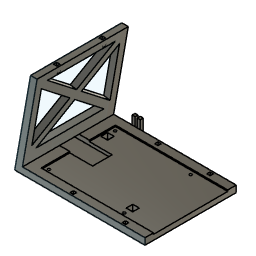
WRO raspberry PI (1) (Autodesk Fusion 360 design; units mm, degrees)
Autodesk Fusion 360 part; units mm, degrees
note: some values were not read from the file. Set by a fixed rule: which sketch regions a step uses.
sketch "Sketch1" plane through (0, 0, 0) normal (0, 1, 0) x (1, 0, 0)
  line L0 (0, 0) -> (12.1554, -68.9365)
  line L1 (0, 0) -> (70, 0) construction
  line L2 (0, 0) -> (100, 0)
  line L3 (100, 0) -> (100, -5)
  line L4 (100, -5) -> (0.8816, -5)
  line L5 (6.0777, -34.4683) -> (10.7761, -32.7582)
  line L6 (6.0777, -34.4683) -> (11.0777, -34.4683) construction
  line L7 (4.1331, -23.4398) -> (8.8315, -21.7297)
  line L8 (4.1331, -23.4398) -> (9.1331, -23.4398) construction
  line L9 (8.8315, -21.7297) -> (10.7761, -32.7582)
  line L10 (10.7761, -32.7582) -> (5, 0)
  line L11 (5, 0) -> (16.8803, -67.3767)
  line L12 (12.1554, -68.9365) -> (20.8902, -68.9365)
  line L13 (16.8803, -67.3767) -> (17.1554, -68.9365)
  dimension "d1" = 70
  dimension "d2" = 80
  dimension "d3" = 100
  dimension "d4" = 5
  dimension "d5" = 5
  dimension "d6" = 20
  dimension "d7" = 20
  dimension "d8" = 5
  constraint horizontal L1
  constraint coincident L0.start L1.start
  constraint parallel L1 L2
  constraint perpendicular L2 L3
  constraint coincident L0 L4.end
  constraint perpendicular L3 L4
  constraint horizontal L6
  constraint midpoint L0 L5.start
  constraint horizontal L8
  constraint coincident L0 L7.start
  constraint coincident L2 L10.end
  constraint parallel L10 L11
  constraint horizontal L12
  constraint coincident L12 L13.end
  constraint parallel L11 L13
  measures "d1" distance of L0.start L0.end
  measures "d2" angle of L0 L1
  measures "d3" distance of L0.start L2.end
  measures "d4" distance of L2.end L3.end
  measures "d5" distance of L5.start L5.end
  measures "d6" angle of L5 L6
  measures "d7" angle of L7 L8
  measures "d8" distance of L7.start L7.end
extrude "Extrude1" add sketch "Sketch1" along normal blind 70 makes body 1
sketch "Sketch2" plane through (0, 0, 0) normal (0, 0, -1) x (1, 0, 0)
  line L0 (100, 0) -> (0, 0)
  line L1 (0, 0) -> (0, -70)
  line L2 (0, -70) -> (100, -70)
  line L3 (100, -70) -> (100, 0)
  line L4 (0, 0) -> (1.25, 0)
  line L5 (1.25, 0) -> (1.25, -1.25)
  line L6 (1.25, -1.25) -> (0, -1.25)
  line L7 (0, -1.25) -> (0, 0)
  line L8 (1.25, -1.25) -> (3.55, -1.25)
  line L9 (3.55, -1.25) -> (3.55, -3.55)
  line L10 (3.55, -3.55) -> (1.25, -3.55)
  line L11 (1.25, -3.55) -> (1.25, -1.25)
  line L12 (0, -70) -> (1.25, -70)
  line L13 (1.25, -70) -> (1.25, -68.75)
  line L14 (1.25, -68.75) -> (0, -68.75)
  line L15 (0, -68.75) -> (0, -70)
  line L16 (1.25, -68.75) -> (3.55, -68.75)
  line L17 (3.55, -68.75) -> (3.55, -66.45)
  line L18 (3.55, -66.45) -> (1.25, -66.45)
  line L19 (1.25, -66.45) -> (1.25, -68.75)
  dimension "d11" = 1.25
  dimension "d12" = 1.25
  dimension "d13" = 2.3
  dimension "d14" = 2.3
  dimension "d15" = 1.25
  dimension "d16" = 1.25
  dimension "d17" = 2.3
  dimension "d18" = 2.3
  constraint horizontal L4
  constraint vertical L5
  constraint horizontal L6
  constraint vertical L7
  constraint coincident L0.end L1.start
  constraint horizontal L8
  constraint vertical L9
  constraint horizontal L10
  constraint vertical L11
  constraint horizontal L12
  constraint vertical L13
  constraint horizontal L14
  constraint vertical L15
  constraint coincident L1.end L2.start
  constraint horizontal L16
  constraint vertical L17
  constraint horizontal L18
  constraint vertical L19
  measures "d11" distance of L0.end L4.end
  measures "d12" distance of L0.end L6.end
  measures "d13" distance of L5.end L8.end
  measures "d14" distance of L5.end L10.end
  measures "d15" distance of L1.end L12.end
  measures "d16" distance of L1.end L14.end
  measures "d17" distance of L13.end L16.end
  measures "d18" distance of L13.end L18.end
extrude "Extrude2" add sketch "Sketch2" along normal blind 5 contours L8 L9 L10 L11 | L16 L17 L18 L19 bodies 1
sketch "Sketch3" plane through (0, 0, 5) normal (0, 0, 1) x (-1, 0, 0)
  line L0 (-5.8816, 0) -> (-100, 0)
  line L1 (-100, 0) -> (-100, -70)
  line L2 (-100, -70) -> (-5.8816, -70)
  line L3 (-5.8816, -70) -> (-5.8816, 0)
  line L4 (-100, 0) -> (-100, -35)
  line L5 (-100, -35) -> (-100, -6.5)
  line L6 (-100, -6.5) -> (-13.75, -6.5)
  line L7 (-13.75, -6.5) -> (-13.75, -63.5)
  line L8 (-13.75, -63.5) -> (-100, -63.5)
  line L9 (-100, -63.5) -> (-100, -6.5)
  dimension "d21" = 35
  dimension "d22" = 28.5
  dimension "d23" = 86.25
  dimension "d24" = 57
  constraint coincident L0.end L1.start
  constraint perpendicular L0 L4
  constraint parallel L4 L5
  constraint horizontal L6
  constraint vertical L7
  constraint horizontal L8
  constraint vertical L9
  measures "d21" distance of L0.end L4.end
  measures "d22" distance of L4.end L5.end
  measures "d23" distance of L5.end L6.end
  measures "d24" distance of L5.end L8.end
extrude "Extrude3" cut sketch "Sketch3" against normal blind 1 contours L1 L4 L5 L6 L7 L8 L9 bodies 1
sketch "Sketch4" plane through (0, 0, 4) normal (0, 0, 1) x (-1, 0, 0)
  line L0 (-100, -63.5) -> (-13.75, -63.5)
  line L1 (-13.75, -63.5) -> (-13.75, -6.5)
  line L2 (-13.75, -6.5) -> (-100, -6.5)
  line L3 (-100, -6.5) -> (-100, -63.5)
  line L4 (-13.75, -6.5) -> (-13.75, -28.5)
  line L5 (-13.75, -28.5) -> (-31.25, -28.5)
  line L6 (-31.25, -28.5) -> (-31.25, -43.5)
  line L7 (-31.25, -43.5) -> (-13.75, -43.5)
  line L8 (-13.75, -43.5) -> (-13.75, -28.5)
  dimension "d27" = 22
  dimension "d28" = 17.5
  dimension "d29" = 15
  constraint coincident L1.end L2.start
  constraint perpendicular L2 L4
  constraint horizontal L5
  constraint vertical L6
  constraint horizontal L7
  constraint vertical L8
  measures "d27" distance of L1.end L4.end
  measures "d28" distance of L4.end L5.end
  measures "d29" distance of L4.end L7.end
extrude "Extrude4" cut sketch "Sketch4" against normal blind 2.5 contours L1 L5 L6 L7 L8 bodies 1
sketch "Sketch5" plane through (13.75, 0, 0) normal (1, 0, 0) x (0, 1, 0)
  line L0 (63.5, 5) -> (6.5, 5)
  line L1 (6.5, 5) -> (6.5, 4)
  line L2 (6.5, 4) -> (28.5, 4)
  line L3 (28.5, 4) -> (28.5, 1.5)
  line L4 (28.5, 1.5) -> (43.5, 1.5)
  line L5 (43.5, 1.5) -> (43.5, 4)
  line L6 (43.5, 4) -> (63.5, 4)
  line L7 (63.5, 4) -> (63.5, 5)
  line L8 (28.5, 1.5) -> (43.5, 1.5)
  line L9 (43.5, 1.5) -> (43.5, 5)
  line L10 (43.5, 5) -> (28.5, 5)
  line L11 (28.5, 5) -> (28.5, 1.5)
  dimension "d32" = 3.5
  constraint horizontal L8
  constraint vertical L9
  constraint horizontal L10
  constraint vertical L11
  constraint coincident L3.end L4.start
  measures "d32" distance of L3.end L10.end
extrude "Extrude5" cut sketch "Sketch5" against normal blind 1000 contours L0 L3 L4 L5 L8 L9 L10 L11 bodies 1
sketch "Sketch6" plane through (0, 0, 4) normal (0, 0, 1) x (-1, 0, 0)
  line L0 (-13.75, -43.5) -> (-31.25, -43.5)
  line L1 (-31.25, -43.5) -> (-31.25, -28.5)
  line L2 (-31.25, -28.5) -> (-13.75, -28.5)
  line L3 (-13.75, -28.5) -> (-13.75, -6.5)
  line L4 (-13.75, -6.5) -> (-100, -6.5)
  line L5 (-100, -6.5) -> (-100, -63.5)
  line L6 (-100, -63.5) -> (-13.75, -63.5)
  line L7 (-13.75, -63.5) -> (-13.75, -43.5)
  line L8 (-13.75, -63.5) -> (-16.55, -63.5)
  line L9 (-16.55, -63.5) -> (-16.55, -60.5)
  circle A0 centre (-16.55, -60.5) radius 1
  dimension "d35" = 2.8
  dimension "d36" = 3
  dimension "d37" = 2
  constraint coincident L6.end L7.start
  constraint perpendicular L7 L8
  constraint perpendicular L6 L9
  constraint coincident L9.end A0.centre
  measures "d35" distance of L6.end L8.end
  measures "d36" distance of L8.end L9.end
  measures "d37" diameter of A0
extrude "Extrude6" cut sketch "Sketch6" against normal blind 67 contours A0 bodies 1
sketch "Sketch7" plane through (0, 0, 4) normal (0, 0, 1) x (-1, 0, 0)
  circle A0 centre (-16.55, -60.5) radius 1
  line L0 (-13.75, -43.5) -> (-31.25, -43.5)
  line L1 (-31.25, -43.5) -> (-31.25, -28.5)
  line L2 (-31.25, -28.5) -> (-13.75, -28.5)
  line L3 (-13.75, -28.5) -> (-13.75, -6.5)
  line L4 (-13.75, -6.5) -> (-100, -6.5)
  line L5 (-100, -6.5) -> (-100, -63.5)
  line L6 (-100, -63.5) -> (-13.75, -63.5)
  line L7 (-13.75, -63.5) -> (-13.75, -43.5)
  line L8 (-16.55, -60.5) -> (-16.55, -59.5)
  line L9 (-16.55, -59.5) -> (-16.55, -56.5)
  line L10 (-16.55, -56.5) -> (-14.75, -56.5)
  line L11 (-14.75, -56.5) -> (-19.75, -56.5)
  line L12 (-19.75, -56.5) -> (-19.75, -51.5)
  line L13 (-19.75, -51.5) -> (-14.75, -51.5)
  line L14 (-14.75, -51.5) -> (-14.75, -56.5)
  dimension "d40" = 3
  dimension "d41" = 1.8
  dimension "d42" = 5
  dimension "d43" = 5
  constraint coincident A0.centre L8.start
  constraint coincident A0 L8.end
  constraint vertical L8
  constraint parallel L8 L9
  constraint perpendicular L7 L10
  constraint horizontal L11
  constraint vertical L12
  constraint horizontal L13
  constraint vertical L14
  measures "d40" distance of L8.end L9.end
  measures "d41" distance of L9.end L10.end
  measures "d42" distance of L10.end L11.end
  measures "d43" distance of L10.end L13.end
extrude "Extrude7" cut sketch "Sketch7" against normal blind 56 contours L10 L11 L12 L13 L14 bodies 1
sketch "Sketch8" plane through (0, 0, 4) normal (0, 0, 1) x (-1, 0, 0)
  line L0 (-19.75, -56.5) -> (-19.75, -51.5)
  line L1 (-19.75, -51.5) -> (-14.75, -51.5)
  line L2 (-14.75, -51.5) -> (-14.75, -56.5)
  line L3 (-14.75, -56.5) -> (-19.75, -56.5)
  circle A0 centre (-16.55, -60.5) radius 1
  line L4 (-13.75, -43.5) -> (-31.25, -43.5)
  line L5 (-31.25, -43.5) -> (-31.25, -28.5)
  line L6 (-31.25, -28.5) -> (-13.75, -28.5)
  line L7 (-13.75, -28.5) -> (-13.75, -6.5)
  line L8 (-13.75, -6.5) -> (-100, -6.5)
  line L9 (-100, -6.5) -> (-100, -63.5)
  line L10 (-100, -63.5) -> (-13.75, -63.5)
  line L11 (-13.75, -63.5) -> (-13.75, -43.5)
  line L12 (-13.75, -6.5) -> (-16.75, -6.5)
  line L13 (-16.75, -6.5) -> (-16.75, -9.5)
  circle A1 centre (-16.75, -9.5) radius 1
  dimension "d46" = 3
  dimension "d47" = 3
  dimension "d48" = 2
  constraint coincident L7.end L8.start
  constraint perpendicular L7 L12
  constraint perpendicular L12 L13
  constraint coincident L13.end A1.centre
  measures "d46" distance of L7.end L12.end
  measures "d47" distance of L12.end L13.end
  measures "d48" diameter of A1
extrude "Extrude8" cut sketch "Sketch8" against normal blind 45 contours A1 bodies 1
sketch "Sketch9" plane through (0, 0, 4) normal (0, 0, 1) x (-1, 0, 0)
  circle A0 centre (-16.75, -9.5) radius 1
  line L0 (-19.75, -56.5) -> (-19.75, -51.5)
  line L1 (-19.75, -51.5) -> (-14.75, -51.5)
  line L2 (-14.75, -51.5) -> (-14.75, -56.5)
  line L3 (-14.75, -56.5) -> (-19.75, -56.5)
  circle A1 centre (-16.55, -60.5) radius 1
  line L4 (-13.75, -43.5) -> (-31.25, -43.5)
  line L5 (-31.25, -43.5) -> (-31.25, -28.5)
  line L6 (-31.25, -28.5) -> (-13.75, -28.5)
  line L7 (-13.75, -28.5) -> (-13.75, -6.5)
  line L8 (-13.75, -6.5) -> (-100, -6.5)
  line L9 (-100, -6.5) -> (-100, -63.5)
  line L10 (-100, -63.5) -> (-13.75, -63.5)
  line L11 (-13.75, -63.5) -> (-13.75, -43.5)
  line L12 (-16.55, -60.5) -> (-74.55, -60.5)
  circle A2 centre (-74.55, -60.5) radius 1
  line L13 (-74.55, -60.5) -> (-74.55, -9.5)
  circle A3 centre (-74.55, -9.5) radius 1
  dimension "d51" = 58
  dimension "d52" = 2
  dimension "d53" = 51
  dimension "d54" = 2
  constraint coincident A1.centre L12.start
  constraint perpendicular L11 L12
  constraint coincident L12.end A2.centre
  constraint vertical L13
  constraint coincident L13.end A3.centre
  measures "d51" distance of A1.centre L12.end
  measures "d52" diameter of A2
  measures "d53" distance of L12.end L13.end
  measures "d54" diameter of A3
extrude "Extrude9" cut sketch "Sketch9" against normal blind 5 contours L12 A2 L13 | L12 A2 L13 | A3 bodies 1
sketch "Sketch10" plane through (0, 0, 4) normal (0, 0, 1) x (-1, 0, 0)
  circle A0 centre (-74.55, -60.5) radius 1
  circle A1 centre (-74.55, -9.5) radius 1
  circle A2 centre (-16.75, -9.5) radius 1
  line L0 (-19.75, -56.5) -> (-19.75, -51.5)
  line L1 (-19.75, -51.5) -> (-14.75, -51.5)
  line L2 (-14.75, -51.5) -> (-14.75, -56.5)
  line L3 (-14.75, -56.5) -> (-19.75, -56.5)
  circle A3 centre (-16.55, -60.5) radius 1
  line L4 (-13.75, -43.5) -> (-31.25, -43.5)
  line L5 (-31.25, -43.5) -> (-31.25, -28.5)
  line L6 (-31.25, -28.5) -> (-13.75, -28.5)
  line L7 (-13.75, -28.5) -> (-13.75, -6.5)
  line L8 (-13.75, -6.5) -> (-100, -6.5)
  line L9 (-100, -6.5) -> (-100, -63.5)
  line L10 (-100, -63.5) -> (-13.75, -63.5)
  line L11 (-13.75, -63.5) -> (-13.75, -43.5)
  line L12 (-74.55, -9.5) -> (-74.55, -13.5)
  line L13 (-74.55, -13.5) -> (-77.05, -13.5)
  line L14 (-77.05, -13.5) -> (-77.05, -18.5)
  line L15 (-77.05, -18.5) -> (-74.55, -18.5)
  line L16 (-74.55, -18.5) -> (-74.55, -13.5)
  line L17 (-77.05, -18.5) -> (-72.05, -18.5)
  line L18 (-72.05, -18.5) -> (-72.05, -13.5)
  line L19 (-72.05, -13.5) -> (-77.05, -13.5)
  line L20 (-77.05, -13.5) -> (-77.05, -18.5)
  dimension "d57" = 4
  dimension "d58" = 2.5
  dimension "d59" = 5
  dimension "d60" = 5
  dimension "d61" = 5
  constraint coincident A1.centre L12.start
  constraint vertical L12
  constraint horizontal L13
  constraint vertical L14
  constraint horizontal L15
  constraint vertical L16
  constraint horizontal L17
  constraint vertical L18
  constraint horizontal L19
  constraint vertical L20
  measures "d57" distance of A1.centre L12.end
  measures "d58" distance of L12.end L13.end
  measures "d59" distance of L12.end L15.end
  measures "d60" distance of L14.end L17.end
  measures "d61" distance of L14.end L13.end
extrude "Extrude10" cut sketch "Sketch10" against normal blind 5 contours L13 L14 L15 L16 L17 L19 L20 | L16 L17 L18 L19 bodies 1
sketch "Sketch11" plane through (0, 0, 0) normal (-0.984808, 0, 0.173648) x (0, -1, 0)
  line L0 (-28.5, 1.5231) -> (-43.5, 1.5231)
  line L1 (-43.5, 1.5231) -> (-43.5, 5.0771)
  line L2 (-43.5, 5.0771) -> (-28.5, 5.0771)
  line L3 (-28.5, 5.0771) -> (-28.5, 1.5231)
  line L4 (0, 0) -> (0, 70)
  line L5 (0, 70) -> (-70, 70)
  line L6 (-70, 70) -> (-70, 0)
  line L7 (-70, 0) -> (0, 0)
sketch "Sketch12" plane through (0, 0, 0) normal (-0.984808, 0, 0.173648) x (0, -1, 0)
  line L0 (-70, 70) -> (0, 70)
  line L1 (0, 70) -> (0, 10)
  line L2 (0, 10) -> (-70, 10)
  line L3 (-70, 10) -> (-70, 70)
  line L4 (-70, 70) -> (-65, 70)
  line L5 (-65, 70) -> (-65, 65)
  line L6 (-65, 65) -> (-5, 65)
  line L7 (-5, 65) -> (-5, 15)
  line L8 (-5, 15) -> (-65, 15)
  line L9 (-65, 15) -> (-65, 65)
  line L10 (-65, 15) -> (-65, 19)
  line L11 (-65, 15) -> (-61, 15)
  line L12 (-5, 65) -> (-9, 65)
  line L13 (-5, 65) -> (-5, 61)
  line L14 (-65, 19) -> (-9, 65)
  line L15 (-5, 61) -> (-61, 15)
  line L16 (-65, 65) -> (-65, 61)
  line L17 (-65, 65) -> (-61, 65)
  line L18 (-5, 15) -> (-5, 19)
  line L19 (-5, 15) -> (-9, 15)
  line L20 (-9, 15) -> (-65, 61)
  line L21 (-5, 19) -> (-61, 65)
  dimension "d64" = 70
  dimension "d65" = 60
  dimension "d66" = 5
  dimension "d67" = 5
  dimension "d68" = 60
  dimension "d69" = 50
  dimension "d70" = 4
  dimension "d71" = 4
  dimension "d72" = 4
  dimension "d73" = 4
  dimension "d74" = 4
  dimension "d75" = 4
  dimension "d76" = 4
  dimension "d77" = 4
  constraint horizontal L0
  constraint vertical L1
  constraint horizontal L2
  constraint vertical L3
  constraint perpendicular L3 L4
  constraint perpendicular L4 L5
  constraint horizontal L6
  constraint vertical L7
  constraint horizontal L8
  constraint vertical L9
  constraint perpendicular L8 L10
  constraint perpendicular L10 L11
  constraint coincident L6 L12.end
  constraint perpendicular L6 L13
  constraint perpendicular L6 L16
  constraint perpendicular L16 L17
  constraint perpendicular L8 L18
  constraint perpendicular L18 L19
  measures "d64" distance of L0.start L0.end
  measures "d65" distance of L0.start L2.end
  measures "d66" distance of L0.start L4.end
  measures "d67" distance of L4.end L5.end
  measures "d68" distance of L5.end L6.end
  measures "d69" distance of L5.end L8.end
  measures "d70" distance of L8.end L10.end
  measures "d71" distance of L8.end L11.end
  measures "d72" distance of L6.end L12.end
  measures "d73" distance of L6.end L13.end
  measures "d74" distance of L5.end L16.end
  measures "d75" distance of L5.end L17.end
  measures "d76" distance of L7.end L18.end
  measures "d77" distance of L7.end L19.end
extrude "Extrude11" cut sketch "Sketch12" against normal blind 5 contours L6 L14 L21 | L9 L14 L20 | L7 L15 L21 | L8 L15 L20 bodies 1
sketch "Sketch13" plane through (0, 0, 68.9365) normal (0, 0, 1) x (-1, 0, 0)
  line L0 (-12.1554, 0) -> (-17.1554, 0)
  line L1 (-17.1554, 0) -> (-17.1554, -70)
  line L2 (-17.1554, -70) -> (-12.1554, -70)
  line L3 (-12.1554, -70) -> (-12.1554, 0)
  line L4 (-12.1554, 0) -> (-12.1554, -35)
  line L5 (-12.1554, -35) -> (-12.1554, -15)
  line L6 (-12.1554, -15) -> (-12.1554, -55)
  line L7 (-12.1554, -55) -> (-17.1554, -55)
  line L8 (-17.1554, -55) -> (-17.1554, -15)
  line L9 (-17.1554, -15) -> (-12.1554, -15)
  line L10 (-12.1554, -15) -> (-12.1554, -55)
  line L11 (-17.1554, -55) -> (-17.1554, -53.65)
  line L12 (-17.1554, -53.65) -> (-15.8054, -53.65)
  line L13 (-15.8054, -53.65) -> (-13.5054, -53.65)
  line L14 (-13.5054, -53.65) -> (-13.5054, -51.35)
  line L15 (-13.5054, -51.35) -> (-15.8054, -51.35)
  line L16 (-15.8054, -51.35) -> (-15.8054, -53.65)
  line L17 (-12.1554, -15) -> (-12.1554, -16.35)
  line L18 (-12.1554, -16.35) -> (-13.5054, -16.35)
  line L19 (-13.5054, -16.35) -> (-15.8054, -16.35)
  line L20 (-15.8054, -16.35) -> (-15.8054, -18.65)
  line L21 (-15.8054, -18.65) -> (-13.5054, -18.65)
  line L22 (-13.5054, -18.65) -> (-13.5054, -16.35)
  dimension "d80" = 35
  dimension "d81" = 20
  dimension "d82" = 40
  dimension "d83" = 5
  dimension "d84" = 40
  dimension "d85" = 1.35
  dimension "d86" = 1.35
  dimension "d87" = 2.3
  dimension "d88" = 2.3
  dimension "d89" = 1.35
  dimension "d90" = 1.35
  dimension "d91" = 2.3
  dimension "d92" = 2.3
  constraint coincident L0.start L3.end
  constraint perpendicular L2 L4
  constraint parallel L4 L5
  constraint parallel L3 L6
  constraint horizontal L7
  constraint vertical L8
  constraint horizontal L9
  constraint vertical L10
  constraint perpendicular L7 L11
  constraint perpendicular L8 L12
  constraint horizontal L13
  constraint vertical L14
  constraint horizontal L15
  constraint vertical L16
  constraint parallel L6 L17
  constraint perpendicular L5 L18
  constraint horizontal L19
  constraint vertical L20
  constraint horizontal L21
  constraint vertical L22
  measures "d80" distance of L0.start L4.end
  measures "d81" distance of L4.end L5.end
  measures "d82" distance of L5.end L6.end
  measures "d83" distance of L6.end L7.end
  measures "d84" distance of L6.end L5.end
  measures "d85" distance of L7.end L11.end
  measures "d86" distance of L11.end L12.end
  measures "d87" distance of L12.end L13.end
  measures "d88" distance of L12.end L15.end
  measures "d89" distance of L5.end L17.end
  measures "d90" distance of L17.end L18.end
  measures "d91" distance of L18.end L19.end
  measures "d92" distance of L18.end L21.end
extrude "Extrude12" cut sketch "Sketch13" against normal blind 5 contours L13 L14 L15 L16 | L19 L20 L21 L22 bodies 1
sketch "Sketch14" plane through (0, 0, 0) normal (0, -1, 0) x (1, 0, 0)
  line L0 (12.1554, 68.9365) -> (0, 0)
  line L1 (0, 0) -> (100, 0)
  line L2 (100, 0) -> (100, 5)
  line L3 (100, 5) -> (5.8816, 5)
  line L4 (5.8816, 5) -> (17.1554, 68.9365)
  line L5 (17.1554, 68.9365) -> (12.1554, 68.9365)
sketch "Sketch15" plane through (0, 0, 68.9365) normal (0, 0, 1) x (-1, 0, 0)
  line L0 (-15.8054, -16.35) -> (-13.5054, -16.35)
  line L1 (-13.5054, -16.35) -> (-13.5054, -18.65)
  line L2 (-13.5054, -18.65) -> (-15.8054, -18.65)
  line L3 (-15.8054, -18.65) -> (-15.8054, -16.35)
  line L4 (-13.5054, -53.65) -> (-15.8054, -53.65)
  line L5 (-15.8054, -53.65) -> (-15.8054, -51.35)
  line L6 (-15.8054, -51.35) -> (-13.5054, -51.35)
  line L7 (-13.5054, -51.35) -> (-13.5054, -53.65)
  line L8 (-12.1554, 0) -> (-17.1554, 0)
  line L9 (-17.1554, 0) -> (-17.1554, -70)
  line L10 (-17.1554, -70) -> (-12.1554, -70)
  line L11 (-12.1554, -70) -> (-12.1554, 0)
  line L12 (-13.5054, -16.35) -> (-13.4054, -16.35)
  line L13 (-13.4054, -16.35) -> (-13.4054, -16.25)
  line L14 (-13.4054, -16.25) -> (-15.9054, -16.25)
  line L15 (-15.9054, -16.25) -> (-15.9054, -18.75)
  line L16 (-15.9054, -18.75) -> (-13.4054, -18.75)
  line L17 (-13.4054, -18.75) -> (-13.4054, -16.25)
  line L18 (-15.8054, -51.35) -> (-15.9054, -51.35)
  line L19 (-15.9054, -51.35) -> (-15.9054, -51.25)
  line L20 (-15.9054, -51.25) -> (-13.4054, -51.25)
  line L21 (-13.4054, -51.25) -> (-13.4054, -53.75)
  line L22 (-13.4054, -53.75) -> (-15.9054, -53.75)
  line L23 (-15.9054, -53.75) -> (-15.9054, -51.25)
  dimension "d95" = 0.1
  dimension "d96" = 0.1
  dimension "d97" = 2.5
  dimension "d98" = 2.5
  dimension "d99" = 0.1
  dimension "d100" = 0.1
  dimension "d101" = 2.5
  dimension "d102" = 2.5
  constraint coincident L0.end L1.start
  constraint horizontal L12
  constraint perpendicular L12 L13
  constraint horizontal L14
  constraint vertical L15
  constraint horizontal L16
  constraint vertical L17
  constraint coincident L5.end L6.start
  constraint horizontal L18
  constraint perpendicular L18 L19
  constraint horizontal L20
  constraint vertical L21
  constraint horizontal L22
  constraint vertical L23
  measures "d95" distance of L0.end L12.end
  measures "d96" distance of L12.end L13.end
  measures "d97" distance of L13.end L14.end
  measures "d98" distance of L13.end L16.end
  measures "d99" distance of L5.end L18.end
  measures "d100" distance of L18.end L19.end
  measures "d101" distance of L19.end L20.end
  measures "d102" distance of L19.end L22.end
extrude "Extrude13" cut sketch "Sketch15" against normal blind 5 contours L13 L14 L15 L16 L17 | L19 L20 L21 L22 L23 bodies 1
sketch "Sketch16" plane through (0, 0, 0) normal (0, 0, -1) x (1, 0, 0)
  line L0 (77.05, -18.5) -> (72.05, -18.5)
  line L1 (72.05, -18.5) -> (72.05, -13.5)
  line L2 (72.05, -13.5) -> (77.05, -13.5)
  line L3 (77.05, -13.5) -> (77.05, -18.5)
  circle A0 centre (74.55, -60.5) radius 1
  circle A1 centre (74.55, -9.5) radius 1
  circle A2 centre (16.75, -9.5) radius 1
  line L4 (19.75, -51.5) -> (19.75, -56.5)
  line L5 (19.75, -56.5) -> (14.75, -56.5)
  line L6 (14.75, -56.5) -> (14.75, -51.5)
  line L7 (14.75, -51.5) -> (19.75, -51.5)
  circle A3 centre (16.55, -60.5) radius 1
  line L8 (1.25, -66.45) -> (3.55, -66.45)
  line L9 (3.55, -66.45) -> (3.55, -68.75)
  line L10 (3.55, -68.75) -> (1.25, -68.75)
  line L11 (1.25, -68.75) -> (1.25, -66.45)
  line L12 (1.25, -3.55) -> (1.25, -1.25)
  line L13 (1.25, -1.25) -> (3.55, -1.25)
  line L14 (3.55, -1.25) -> (3.55, -3.55)
  line L15 (3.55, -3.55) -> (1.25, -3.55)
  line L16 (100, 0) -> (0, 0)
  line L17 (0, 0) -> (0, -70)
  line L18 (0, -70) -> (100, -70)
  line L19 (100, -70) -> (100, 0)
  line L20 (0, 0) -> (5, 0)
  line L21 (5, 0) -> (40, 0)
  line L22 (40, 0) -> (45, 0)
  line L23 (45, 0) -> (85, 0)
  line L24 (85, 0) -> (85, -1.25)
  line L25 (85, -1.25) -> (83.75, -1.25)
  line L26 (83.75, -1.25) -> (81.25, -1.25)
  line L27 (81.25, -1.25) -> (81.25, -3.75)
  line L28 (81.25, -3.75) -> (83.75, -3.75)
  line L29 (83.75, -3.75) -> (83.75, -1.25)
  line L30 (40, 0) -> (41.25, 0)
  line L31 (41.25, 0) -> (41.25, -1.25)
  line L32 (41.25, -1.25) -> (40, -1.25)
  line L33 (40, -1.25) -> (40, 0)
  line L34 (41.25, -1.25) -> (43.75, -1.25)
  line L35 (43.75, -1.25) -> (43.75, -3.75)
  line L36 (43.75, -3.75) -> (41.25, -3.75)
  line L37 (41.25, -3.75) -> (41.25, -1.25)
  dimension "d105" = 5
  dimension "d106" = 35
  dimension "d107" = 40
  dimension "d108" = 1.25
  dimension "d109" = 1.25
  dimension "d110" = 2.5
  dimension "d111" = 2.5
  dimension "d112" = 1.25
  dimension "d113" = 1.25
  dimension "d114" = 2.5
  dimension "d115" = 2.5
  constraint coincident L16.end L17.start
  constraint perpendicular L17 L20
  constraint parallel L16 L21
  constraint coincident L16 L22.end
  constraint parallel L16 L22
  constraint parallel L16 L23
  constraint perpendicular L23 L24
  constraint perpendicular L24 L25
  constraint horizontal L26
  constraint vertical L27
  constraint horizontal L28
  constraint vertical L29
  constraint horizontal L30
  constraint vertical L31
  constraint horizontal L32
  constraint vertical L33
  constraint horizontal L34
  constraint vertical L35
  constraint horizontal L36
  constraint vertical L37
  measures "d105" distance of L16.end L20.end
  measures "d106" distance of L20.end L21.end
  measures "d107" distance of L22.end L23.end
  measures "d108" distance of L23.end L24.end
  measures "d109" distance of L24.end L25.end
  measures "d110" distance of L25.end L26.end
  measures "d111" distance of L25.end L28.end
  measures "d112" distance of L21.end L30.end
  measures "d113" distance of L21.end L32.end
  measures "d114" distance of L31.end L34.end
  measures "d115" distance of L31.end L36.end
extrude "Extrude14" cut sketch "Sketch16" against normal blind 5 contours L34 L35 L36 L37 | L26 L27 L28 L29 bodies 1
sketch "Sketch17" plane through (0, 0, 0) normal (0, 0, -1) x (1, 0, 0)
  line L0 (81.25, -1.25) -> (83.75, -1.25)
  line L1 (83.75, -1.25) -> (83.75, -3.75)
  line L2 (83.75, -3.75) -> (81.25, -3.75)
  line L3 (81.25, -3.75) -> (81.25, -1.25)
  line L4 (43.75, -1.25) -> (43.75, -3.75)
  line L5 (43.75, -3.75) -> (41.25, -3.75)
  line L6 (41.25, -3.75) -> (41.25, -1.25)
  line L7 (41.25, -1.25) -> (43.75, -1.25)
  line L8 (77.05, -18.5) -> (72.05, -18.5)
  line L9 (72.05, -18.5) -> (72.05, -13.5)
  line L10 (72.05, -13.5) -> (77.05, -13.5)
  line L11 (77.05, -13.5) -> (77.05, -18.5)
  circle A0 centre (74.55, -60.5) radius 1
  circle A1 centre (74.55, -9.5) radius 1
  circle A2 centre (16.75, -9.5) radius 1
  line L12 (19.75, -51.5) -> (19.75, -56.5)
  line L13 (19.75, -56.5) -> (14.75, -56.5)
  line L14 (14.75, -56.5) -> (14.75, -51.5)
  line L15 (14.75, -51.5) -> (19.75, -51.5)
  circle A3 centre (16.55, -60.5) radius 1
  line L16 (1.25, -66.45) -> (3.55, -66.45)
  line L17 (3.55, -66.45) -> (3.55, -68.75)
  line L18 (3.55, -68.75) -> (1.25, -68.75)
  line L19 (1.25, -68.75) -> (1.25, -66.45)
  line L20 (1.25, -3.55) -> (1.25, -1.25)
  line L21 (1.25, -1.25) -> (3.55, -1.25)
  line L22 (3.55, -1.25) -> (3.55, -3.55)
  line L23 (3.55, -3.55) -> (1.25, -3.55)
  line L24 (100, 0) -> (0, 0)
  line L25 (0, 0) -> (0, -70)
  line L26 (0, -70) -> (100, -70)
  line L27 (100, -70) -> (100, 0)
  line L28 (41.25, -1.25) -> (41.25, -68.75)
  line L29 (41.25, -68.75) -> (43.75, -68.75)
  line L30 (43.75, -68.75) -> (43.75, -66.25)
  line L31 (43.75, -66.25) -> (41.25, -66.25)
  line L32 (41.25, -66.25) -> (41.25, -68.75)
  line L33 (83.75, -1.25) -> (83.75, -68.75)
  line L34 (83.75, -68.75) -> (81.25, -68.75)
  line L35 (81.25, -68.75) -> (81.25, -66.25)
  line L36 (81.25, -66.25) -> (83.75, -66.25)
  line L37 (83.75, -66.25) -> (83.75, -68.75)
  dimension "d118" = 67.5
  dimension "d119" = 2.5
  dimension "d120" = 2.5
  dimension "d121" = 67.5
  dimension "d122" = 2.5
  dimension "d123" = 2.5
  constraint coincident L6.end L7.start
  constraint perpendicular L26 L28
  constraint horizontal L29
  constraint vertical L30
  constraint horizontal L31
  constraint vertical L32
  constraint coincident L0.end L1.start
  constraint perpendicular L26 L33
  constraint horizontal L34
  constraint vertical L35
  constraint horizontal L36
  constraint vertical L37
  measures "d118" distance of L6.end L28.end
  measures "d119" distance of L28.end L29.end
  measures "d120" distance of L28.end L31.end
  measures "d121" distance of L0.end L33.end
  measures "d122" distance of L33.end L34.end
  measures "d123" distance of L33.end L36.end
extrude "Extrude15" cut sketch "Sketch17" against normal blind 5 contours L28 L29 L30 L31 L32 | L33 L34 L35 L36 L37 bodies 1
extrude "Extrude16" cut 2 faces at (2.0167, 2.0167, -5) (2.0167, 67.2167, -5) along direction (0, 0, 1) blind 10 on bodies 1 bodies 1
sketch "Sketch18" plane through (0, 0, 0) normal (0, 0, 1) x (1, 0, 0)
  line L0 (24.7547, 77.5718) -> (22.4547, 77.5718)
  line L1 (22.4547, 77.5718) -> (22.4547, 79.8718)
  line L2 (22.4547, 79.8718) -> (24.7547, 79.8718)
  line L3 (24.7547, 79.8718) -> (24.7547, 77.5718)
  dimension "d128" = 2.3
  dimension "d129" = 2.3
  constraint horizontal L0
  constraint vertical L1
  constraint horizontal L2
  constraint vertical L3
  measures "d128" distance of L0.start L0.end
  measures "d129" distance of L0.start L2.end
extrude "Extrude17" add sketch "Sketch18" along normal blind 5 separate body makes body 2
extrude "Extrude18" add 1 faces at (23.988, 78.3385, 5) along direction (0, 0, 1) blind 5 on bodies 2 bodies 2
sketch "Sketch19" plane through (0, 0, 0) normal (0, 0, -1) x (1, 0, 0)
  line L0 (81.25, -68.75) -> (81.25, -66.25)
  line L1 (81.25, -66.25) -> (83.75, -66.25)
  line L2 (83.75, -66.25) -> (83.75, -68.75)
  line L3 (83.75, -68.75) -> (81.25, -68.75)
  line L4 (43.75, -68.75) -> (41.25, -68.75)
  line L5 (41.25, -68.75) -> (41.25, -66.25)
  line L6 (41.25, -66.25) -> (43.75, -66.25)
  line L7 (43.75, -66.25) -> (43.75, -68.75)
  line L8 (81.25, -1.25) -> (83.75, -1.25)
  line L9 (83.75, -1.25) -> (83.75, -3.75)
  line L10 (83.75, -3.75) -> (81.25, -3.75)
  line L11 (81.25, -3.75) -> (81.25, -1.25)
  line L12 (43.75, -1.25) -> (43.75, -3.75)
  line L13 (43.75, -3.75) -> (41.25, -3.75)
  line L14 (41.25, -3.75) -> (41.25, -1.25)
  line L15 (41.25, -1.25) -> (43.75, -1.25)
  line L16 (77.05, -18.5) -> (72.05, -18.5)
  line L17 (72.05, -18.5) -> (72.05, -13.5)
  line L18 (72.05, -13.5) -> (77.05, -13.5)
  line L19 (77.05, -13.5) -> (77.05, -18.5)
  circle A0 centre (74.55, -60.5) radius 1
  circle A1 centre (74.55, -9.5) radius 1
  circle A2 centre (16.75, -9.5) radius 1
  line L20 (19.75, -51.5) -> (19.75, -56.5)
  line L21 (19.75, -56.5) -> (14.75, -56.5)
  line L22 (14.75, -56.5) -> (14.75, -51.5)
  line L23 (14.75, -51.5) -> (19.75, -51.5)
  circle A3 centre (16.55, -60.5) radius 1
  line L24 (1.25, -66.45) -> (3.55, -66.45)
  line L25 (3.55, -66.45) -> (3.55, -68.75)
  line L26 (3.55, -68.75) -> (1.25, -68.75)
  line L27 (1.25, -68.75) -> (1.25, -66.45)
  line L28 (1.25, -3.55) -> (1.25, -1.25)
  line L29 (1.25, -1.25) -> (3.55, -1.25)
  line L30 (3.55, -1.25) -> (3.55, -3.55)
  line L31 (3.55, -3.55) -> (1.25, -3.55)
  line L32 (100, 0) -> (0, 0)
  line L33 (0, 0) -> (0, -70)
  line L34 (0, -70) -> (100, -70)
  line L35 (100, -70) -> (100, 0)
  line L36 (1.25, -1.25) -> (1.25, -1.15)
  line L37 (1.2278, -1.15) -> (1.1278, -1.15)
  line L38 (1.1278, -1.15) -> (3.6278, -1.15)
  line L39 (3.6278, -1.15) -> (3.6278, -3.65)
  line L40 (3.6278, -3.65) -> (1.1278, -3.65)
  line L41 (1.1278, -3.65) -> (1.1278, -1.15)
  dimension "d134" = 0.1
  dimension "d135" = 0.1
  dimension "d136" = 2.5
  dimension "d137" = 2.5
  constraint coincident L28.end L29.start
  constraint vertical L36
  constraint perpendicular L36 L37
  constraint horizontal L38
  constraint vertical L39
  constraint horizontal L40
  constraint vertical L41
  measures "d134" distance of L28.end L36.end
  measures "d135" distance of L37.start L37.end
  measures "d136" distance of L37.end L38.end
  measures "d137" distance of L37.end L40.end
extrude "Extrude19" cut sketch "Sketch19" against normal blind 5 contours L37 L38 L39 L40 L41 bodies 1
sketch "Sketch20" plane through (0, 0, 0) normal (0, 0, -1) x (1, 0, 0)
  line L0 (3.6278, -1.15) -> (3.6278, -3.65)
  line L1 (3.6278, -3.65) -> (1.1278, -3.65)
  line L2 (1.1278, -3.65) -> (1.1278, -1.15)
  line L3 (1.1278, -1.15) -> (3.6278, -1.15)
  line L4 (81.25, -68.75) -> (81.25, -66.25)
  line L5 (81.25, -66.25) -> (83.75, -66.25)
  line L6 (83.75, -66.25) -> (83.75, -68.75)
  line L7 (83.75, -68.75) -> (81.25, -68.75)
  line L8 (43.75, -68.75) -> (41.25, -68.75)
  line L9 (41.25, -68.75) -> (41.25, -66.25)
  line L10 (41.25, -66.25) -> (43.75, -66.25)
  line L11 (43.75, -66.25) -> (43.75, -68.75)
  line L12 (81.25, -1.25) -> (83.75, -1.25)
  line L13 (83.75, -1.25) -> (83.75, -3.75)
  line L14 (83.75, -3.75) -> (81.25, -3.75)
  line L15 (81.25, -3.75) -> (81.25, -1.25)
  line L16 (43.75, -1.25) -> (43.75, -3.75)
  line L17 (43.75, -3.75) -> (41.25, -3.75)
  line L18 (41.25, -3.75) -> (41.25, -1.25)
  line L19 (41.25, -1.25) -> (43.75, -1.25)
  line L20 (77.05, -18.5) -> (72.05, -18.5)
  line L21 (72.05, -18.5) -> (72.05, -13.5)
  line L22 (72.05, -13.5) -> (77.05, -13.5)
  line L23 (77.05, -13.5) -> (77.05, -18.5)
  circle A0 centre (74.55, -60.5) radius 1
  circle A1 centre (74.55, -9.5) radius 1
  circle A2 centre (16.75, -9.5) radius 1
  line L24 (19.75, -51.5) -> (19.75, -56.5)
  line L25 (19.75, -56.5) -> (14.75, -56.5)
  line L26 (14.75, -56.5) -> (14.75, -51.5)
  line L27 (14.75, -51.5) -> (19.75, -51.5)
  circle A3 centre (16.55, -60.5) radius 1
  line L28 (1.25, -66.45) -> (3.55, -66.45)
  line L29 (3.55, -66.45) -> (3.55, -68.75)
  line L30 (3.55, -68.75) -> (1.25, -68.75)
  line L31 (1.25, -68.75) -> (1.25, -66.45)
  line L32 (100, 0) -> (0, 0)
  line L33 (0, 0) -> (0, -70)
  line L34 (0, -70) -> (100, -70)
  line L35 (100, -70) -> (100, 0)
  line L36 (3.55, -68.75) -> (3.65, -68.75)
  line L37 (3.65, -68.75) -> (3.65, -68.85)
  line L38 (3.65, -68.85) -> (1.15, -68.85)
  line L39 (1.15, -68.85) -> (1.15, -66.35)
  line L40 (1.15, -66.35) -> (3.65, -66.35)
  line L41 (3.65, -66.35) -> (3.65, -68.85)
  dimension "d140" = 0.1
  dimension "d141" = 0.1
  dimension "d142" = 2.5
  dimension "d143" = 2.5
  constraint coincident L29.end L30.start
  constraint perpendicular L29 L36
  constraint perpendicular L36 L37
  constraint horizontal L38
  constraint vertical L39
  constraint horizontal L40
  constraint vertical L41
  measures "d140" distance of L29.end L36.end
  measures "d141" distance of L36.end L37.end
  measures "d142" distance of L37.end L38.end
  measures "d143" distance of L37.end L40.end
extrude "Extrude20" cut sketch "Sketch20" against normal blind 5 contours L37 L38 L39 L40 L41 bodies 1
copy_body "CopyPasteBodies1" bodies 2 makes body 3
move_body "Move1" bodies 3 to x (1, 0, 0) y (0, 1, 0) z (0, 0, 1) at (-4, -6, 0)
move_body "Move2" bodies 2 to x (1, 0, 0) y (0, 1, 0) z (0, 0, 1) at (0, -6, 0)
